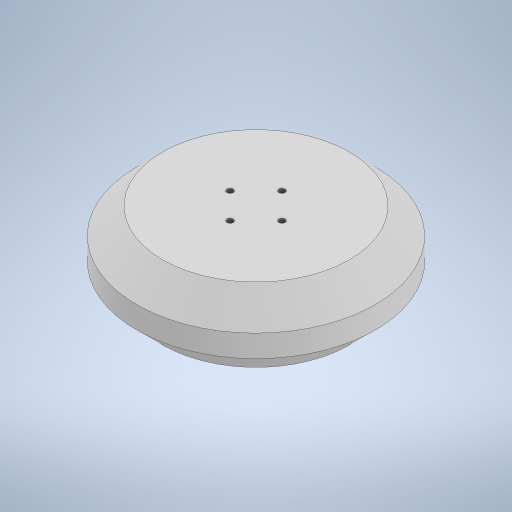
# Autodesk Inventor part: EAGLE POWER 8308
Saved by Autodesk Inventor 2023 (Build 270158030, 158C)
## iProperties
Created: 2022-10-29
Part Number: EAGLE POWER 8308
Material: Generic
Document SubType Name: Modeling
Designer: cjj5381
Density: 1 g/cm^3
Appearance: Default
Author: cjj5381
Autodesk Inventor part; units mm, degrees
ref_plane "YZ Plane" through (0, 0, 0) normal (1, 0, 0) x (0, 1, 0)
ref_plane "XZ Plane" through (0, 0, 0) normal (0, 1, 0) x (-1, 0, 0)
ref_plane "XY Plane" through (0, 0, 0) normal (0, 0, 1) x (1, 0, 0)
sketch "Sketch1" plane through (0, 0, 0) normal (0, 1, 0) x (-1, 0, 0)
  circle A0 centre (0, 0) radius 46
  dimension "d2" = 92
  constraints: 1 centre point, 1 coincident
  measures "d2" diameter of A0
extrude "Extrusion1" add sketch "Sketch1" along normal blind 28.5
chamfer "Chamfer1" distance 10 angle 45 2 edges at (46, 0, 0) (46, 28.5, 0)
sketch "Sketch2" plane through (0, 28.5, 0) normal (0, 1, 0) x (1, 0, 0)
  circle A0 centre (0, 0) radius 36 projected
  circle A1 centre (0, 0) radius 10 construction
  point P0 (-0.4003, 0.0036)
  point P1 (12.4744, -1.9294)
  point P2 (10, 0)
  point P3 (0, -10)
  point P4 (-10, 0)
  point P5 (0, 10)
  dimension "d13" = 20
  constraints: 4 point on circle, 2 coincident, 1 centre point
  measures "d13" diameter of A1
hole "Hole1" at (10, 28.5, 0) at (0, 28.5, 10) at (-10, 28.5, 0) at (0, 28.5, -10) direction (0, -1, 0) diameter 2.459 depth 8.8 tip angle 118 thread size "M3x0.5" class "6H" standard "ISO Metric profile"
sketch "Sketch3" plane through (0, 0, 0) normal (0, -1, 0) x (1, 0, 0)
  circle A0 centre (0, 0) radius 2.5
  dimension "d14" = 5
  constraints: 1 centre point, 1 coincident
  measures "d14" diameter of A0
extrude "Extrusion2" add sketch "Sketch3" along normal blind 5
body "Solid1"
